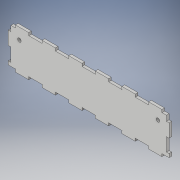
# Autodesk Inventor part: 13 achter plaat LCD
Saved by Autodesk Inventor 2019 (Build 230136000, 136)
## iProperties
Created: 2021-04-20
Part Number: 13 achter plaat LCD
Material: Generic
Document SubType Name: Sheet Metal
Designer: Stefan
Density: 1 g/cm^3
Sheet Metal Rule: Default_mm
Appearance: Default
Author: Stefan
Autodesk Inventor part; units mm, degrees
ref_plane "YZ Plane" through (0, 0, 0) normal (1, 0, 0) x (0, 1, 0)
ref_plane "XZ Plane" through (0, 0, 0) normal (0, 1, 0) x (-1, 0, 0)
ref_plane "XY Plane" through (0, 0, 0) normal (0, 0, 1) x (1, 0, 0)
sketch "Sketch1" plane through (0, 0, 0) normal (0, 0, 1) x (1, 0, 0)
  line L0 (-87.5, -20) -> (87.5, -20)
  line L1 (87.5, -20) -> (87.5, 20)
  line L2 (87.5, 20) -> (-87.5, 20)
  line L3 (-87.5, 20) -> (-87.5, -20)
  line L4 (-87.5, -20) -> (87.5, 20) construction
  line L5 (87.5, -20) -> (-87.5, 20) construction
  line L6 (-87.5, 14) -> (-90.5, 14)
  line L7 (-90.5, 14) -> (-90.5, -1)
  line L8 (-90.5, -1) -> (-87.5, -1)
  line L9 (-87.5, -1) -> (-87.5, 14)
  line L10 (-87.5, -20) -> (-90.5, -20)
  line L11 (-90.5, -20) -> (-90.5, -16)
  line L12 (-90.5, -16) -> (-87.5, -16)
  line L13 (-87.5, -16) -> (-87.5, -20)
  line L14 (0, 20) -> (0, -20) construction
  line L15 (87.5, 14) -> (90.5, 14)
  line L16 (90.5, 14) -> (90.5, -1)
  line L17 (90.5, -1) -> (87.5, -1)
  line L18 (87.5, -1) -> (87.5, 14)
  line L19 (87.5, -20) -> (90.5, -20)
  line L20 (90.5, -20) -> (90.5, -16)
  line L21 (90.5, -16) -> (87.5, -16)
  line L22 (87.5, -16) -> (87.5, -20)
  point P0 (0, 0)
  dimension "d0" = 175
  dimension "d1" = 40
  dimension "d2" = 3
  dimension "d3" = 15
  dimension "d4" = 6
  dimension "d5" = 3
  dimension "d6" = 15
  constraints: 46 end point, 7 symmetric about line, 6 parallel, 4 midpoint, 3 horizontal, 3 perpendicular, 1 point on line
  measures "d0" distance of L2.end L1.end
  measures "d1" distance of L1.end L0.end
  measures "d2" distance of L8.end L7.end
  measures "d3" distance of L7.end L6.end
  measures "d4" distance from line of L2.end L6
  measures "d5" distance of L11.end L12.end
  measures "d6" distance between parallel lines of L8 L12
extrude "Extrusion1" add sketch "Sketch1" along normal blind 3
sketch "Sketch2" plane through (0, 0, 3) normal (0, 0, 1) x (1, 0, 0)
  line L0 (-90.5, -20) -> (90.5, -20)
  line L1 (-82.5, -20) -> (-67.5, -20)
  line L2 (-67.5, -20) -> (-67.5, -23)
  line L3 (-67.5, -23) -> (-82.5, -23)
  line L4 (-82.5, -23) -> (-82.5, -20)
  line L5 (-52.5, -20) -> (-37.5, -20)
  line L6 (-37.5, -20) -> (-37.5, -23)
  line L7 (-37.5, -23) -> (-52.5, -23)
  line L8 (-52.5, -23) -> (-52.5, -20)
  line L9 (-22.5, -20) -> (-7.5, -20)
  line L10 (-7.5, -20) -> (-7.5, -23)
  line L11 (-7.5, -23) -> (-22.5, -23)
  line L12 (-22.5, -23) -> (-22.5, -20)
  line L13 (7.5, -20) -> (22.5, -20)
  line L14 (22.5, -20) -> (22.5, -23)
  line L15 (22.5, -23) -> (7.5, -23)
  line L16 (7.5, -23) -> (7.5, -20)
  line L17 (37.5, -20) -> (52.5, -20)
  line L18 (52.5, -20) -> (52.5, -23)
  line L19 (52.5, -23) -> (37.5, -23)
  line L20 (37.5, -23) -> (37.5, -20)
  line L21 (67.5, -20) -> (82.5, -20)
  line L22 (82.5, -20) -> (82.5, -23)
  line L23 (82.5, -23) -> (67.5, -23)
  line L24 (67.5, -23) -> (67.5, -20)
  line L25 (-82.5, 23) -> (-67.5, 23)
  line L26 (-67.5, 23) -> (-67.5, 20)
  line L27 (-67.5, 20) -> (-82.5, 20)
  line L28 (-82.5, 20) -> (-82.5, 23)
  line L29 (-52.5, 23) -> (-37.5, 23)
  line L30 (-37.5, 23) -> (-37.5, 20)
  line L31 (-37.5, 20) -> (-52.5, 20)
  line L32 (-52.5, 20) -> (-52.5, 23)
  line L33 (-22.5, 23) -> (-7.5, 23)
  line L34 (-7.5, 23) -> (-7.5, 20)
  line L35 (-7.5, 20) -> (-22.5, 20)
  line L36 (-22.5, 20) -> (-22.5, 23)
  line L37 (7.5, 23) -> (22.5, 23)
  line L38 (22.5, 23) -> (22.5, 20)
  line L39 (22.5, 20) -> (7.5, 20)
  line L40 (7.5, 20) -> (7.5, 23)
  line L41 (37.5, 23) -> (52.5, 23)
  line L42 (52.5, 23) -> (52.5, 20)
  line L43 (52.5, 20) -> (37.5, 20)
  line L44 (37.5, 20) -> (37.5, 23)
  line L45 (67.5, 23) -> (82.5, 23)
  line L46 (82.5, 23) -> (82.5, 20)
  line L47 (82.5, 20) -> (67.5, 20)
  line L48 (67.5, 20) -> (67.5, 23)
  line L49 (-90.5, -16) -> (-90.5, -20) projected
  line L50 (-87.5, -16) -> (-90.5, -16) projected
  point P0 (0, 0)
  point P1 (0, 0)
  dimension "d13" = 15
  dimension "d14" = 3
  dimension "d16" = 30
  dimension "d17" = 43
  dimension "d18" = 8
  dimension "d19" = 4
  constraints: 98 end point, 2 horizontal, 2 parallel, 1 collinear, 1 perpendicular, 1 point on line, 1 vertical, 87 other
  measures "d13" distance of L2.end L3.end
  measures "d14" distance of L2.start L2.end
  measures "d16" distance of L1.start L5.start
  measures "d17" distance of L1.start L25.start
  measures "d18" distance between parallel lines of L49 L4
  measures "d19" distance between parallel lines of L50 L0
extrude "Extrusion2" add sketch "Sketch2" against normal blind 3
sketch "Sketch3" plane through (0, 0, 3) normal (0, 0, 1) x (1, 0, 0)
  circle A0 centre (-78, 10.5) radius 2
  circle A1 centre (78, 10.5) radius 2
  line L0 (87.5, 14) -> (87.5, 20) projected
  line L1 (87.5, 20) -> (82.5, 20) projected
  line L2 (-52.5, 20) -> (-67.5, 20) projected
  line L3 (-87.5, 20) -> (-87.5, 14) projected
  point P0 (0, 0)
  dimension "d22" = 4
  dimension "d23" = 4
  dimension "d24" = 9.5
  dimension "d25" = 9.5
  dimension "d26" = 9.5
  dimension "d27" = 9.5
  constraints: 2 centre point
  measures "d22" diameter of A0
  measures "d23" diameter of A1
  measures "d24" distance from line of L0 A1.centre
  measures "d25" distance from line of L1 A1.centre
  measures "d26" distance from line of L2 A0.centre
  measures "d27" distance from line of L3 A0.centre
extrude "Extrusion3" cut sketch "Sketch3" against normal blind 10
equation "\"BendRadius\" = Thickness"
equation "\"BendReliefWidth\" = Thickness"
equation "\"BendReliefDepth\" = 0.5 * Thickness"
equation "\"CornerReliefSize\" = 4 * Thickness"
equation "\"MinimumRemnant\" = 2 * Thickness"
equation "\"TransitionRadius\" = BendRadius"
equation "\"JacobiRadiusSize\" = BendRadius"
equation "\"GapSize\" = Thickness"
equation "\"Thickness\" = 0.5"
body "Solid1"
